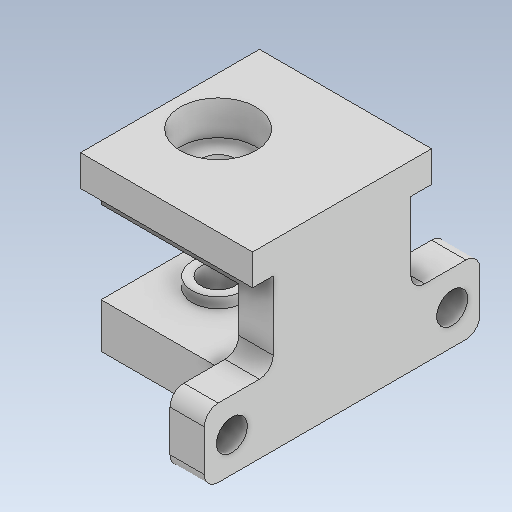
# Autodesk Inventor part: 10-03-024
Saved by Autodesk Inventor 2020 (Build 240168000, 168)
## iProperties
Created: 2019-11-02
Part Number: 10-03-024
Material: Generic
Document SubType Name: Modeling
Designer: iuliu
Density: 1 g/cm^3
Appearance: Default
Description: Intinzator X
Mass: 9.36931 g
Surface Area: 50.6885 cm^2
Volume: 9.36931 cm^3
Author: iuliu
Subject: 012
Autodesk Inventor part; units mm, degrees
ref_plane "YZ Plane" through (0, 0, 0) normal (1, 0, 0) x (0, 1, 0)
ref_plane "XZ Plane" through (0, 0, 0) normal (0, 1, 0) x (-1, 0, 0)
ref_plane "XY Plane" through (0, 0, 0) normal (0, 0, 1) x (1, 0, 0)
sketch "Sketch1" plane through (0, 0, 0) normal (0, 0, 1) x (1, 0, 0)
  line L0 (-12.5, 12.5) -> (12.5, 12.5)
  line L1 (12.5, 12.5) -> (12.5, -12.5)
  line L2 (12.5, -12.5) -> (-12.5, -12.5)
  line L3 (-12.5, -12.5) -> (-12.5, 12.5)
  point P0 (0, 0)
  point P1 (-12.5, 0)
  point P2 (0, 12.5)
  dimension "d0" = 25
  dimension "d1" = 25
  constraints: 8 end point, 2 midpoint, 2 parallel, 1 horizontal, 1 horizontal alignment, 1 perpendicular, 1 vertical alignment
  measures "d0" distance of L2.end L0.start
  measures "d1" distance between parallel lines of L1 L3
extrude "Extrusion1" add sketch "Sketch1" along normal blind 20
sketch "Sketch2" plane through (0, 0, 20) normal (0, 0, 1) x (1, 0, 0)
  line L0 (-12.5, -6) -> (7.5, -6)
  line L1 (7.5, -6) -> (7.5, 6)
  line L2 (7.5, 6) -> (-12.5, 6)
  line L3 (-12.5, 6) -> (-12.5, -6)
  line L4 (-12.5, 12.5) -> (-12.5, -12.5) projected
  line L5 (12.5, -12.5) -> (12.5, 12.5) projected
  point P0 (0, 0)
  point P1 (7.5, 0)
  point P2 (12.5, 0)
  dimension "d4" = 12
  dimension "d5" = 5
  constraints: 8 end point, 2 midpoint, 2 parallel, 1 collinear, 1 horizontal, 1 horizontal alignment, 1 perpendicular
  measures "d4" distance of L0.end L1.end
  measures "d5" distance between parallel lines of L5 L1
extrude "Extrusion2" cut sketch "Sketch2" against normal through all
sketch "Sketch3" plane through (-12.5, -12.5, 0) normal (0, -1, 0) x (1, 0, 0)
  line L0 (0, 0) -> (0, 20) projected
  point P0 (12.5, 0)
  point P1 (7, 10)
  point P2 (0, 10)
  dimension "d8" = 7
  constraints: 1 horizontal alignment, 1 midpoint
  measures "d8" distance from line of L0 point (7, 10)
hole "Hole1" at (-5.5, -12.5, 10) direction (0, 1, 0) diameter 5 end through all
sketch "Sketch4" plane through (-12.5, 12.5, 0) normal (0, 1, 0) x (1, 0, 0)
  line L0 (25, -23) -> (0, -23)
  line L1 (0, -23) -> (0, -20)
  line L2 (0, -20) -> (25, -20)
  line L3 (25, -20) -> (25, -23)
  line L4 (25, -20) -> (0, -20) projected
  line L5 (0, 0) -> (0, -20) projected
  line L6 (25, 0) -> (25, -20) projected
  line L7 (25, 0) -> (0, 0)
  line L8 (0, 0) -> (0, 3)
  line L9 (0, 3) -> (25, 3)
  line L10 (25, 3) -> (25, 0)
  line L11 (25, 0) -> (0, 0) projected
  point P0 (12.5, 0)
  dimension "d16" = 3
  constraints: 16 end point, 7 collinear, 4 parallel, 2 horizontal, 2 perpendicular
  measures "d16" distance of L2.end L0.start
extrude "Extrusion3" add sketch "Sketch4" against normal blind 3 contours L0 L1 L2 L3 | L7 L8 L9 L10
sketch "Sketch7" plane through (12.5, -12.5, 20) normal (1, 0, 0) x (0, 0, -1)
  line L0 (-10, 0) -> (-10, 10)
  line L1 (-10, 10) -> (30, 10)
  line L2 (30, 10) -> (30, 0)
  line L3 (20, 0) -> (0, 0) projected
  line L4 (20, 0) -> (20, 22) projected
  line L5 (0, 0) -> (0, 22) projected
  circle A0 centre (26, 5) radius 2.25
  circle A1 centre (-6, 5) radius 2.25
  line L6 (20, 0) -> (0, 0) projected
  line L7 (-10, 0) -> (32.446, 0)
  point P0 (20, 12.5)
  point P1 (30, 5)
  point P2 (20, 10)
  point P3 (0, 10)
  point P4 (20, 0)
  point P5 (0, 0)
  dimension "d30" = 10
  dimension "d31" = 10
  dimension "d32" = 4.5
  dimension "d33" = 4
  dimension "d34" = 4
  dimension "d50" = 10
  dimension "d51" = 0
  constraints: 8 end point, 2 centre point, 2 horizontal alignment, 1 equal radius, 1 horizontal, 1 midpoint, 1 parallel, 1 point on line
  measures "d30" distance between parallel lines of L4 L2
  measures "d31" distance between parallel lines of L5 L0
  measures "d32" diameter of A0
  measures "d33" distance from line of L2 A0.centre
  measures "d34" distance from line of L0 A1.centre
  measures "d50" distance between parallel lines of L6 L1
  measures "d51" distance between parallel lines of L3 L7
extrude "Extrusion5" add sketch "Sketch7" against normal up to surface (5 mm away) contours L0 L1 L5 L7 | L4 L1 L2 L7
sketch "Sketch6" plane through (-12.5, 12.5, 23) normal (0, 1, 0) x (1, 0, 0)
  circle A0 centre (7, 13) radius 2.5 projected
  circle A1 centre (7, 13) radius 1.5
  point P0 (12.5, 23)
  dimension "d26" = 3
  constraints: 1 centre point, 1 coincident
  measures "d26" diameter of A1
extrude "Extrusion4" add sketch "Sketch6" against normal blind 2
sketch "Sketch8" plane through (-12.5, 12.5, 23) normal (0, 1, 0) x (1, 0, 0)
  circle A0 centre (7, 13) radius 1.5 projected
  circle A1 centre (7, 13) radius 3.75
  point P0 (12.5, 23)
  dimension "d37" = 7.5
  constraints: 1 centre point, 1 coincident
  measures "d37" diameter of A1
extrude "Extrusion6" add sketch "Sketch8" against normal up to surface (25 mm away)
sketch "Sketch9" plane through (-12.5, 12.5, 23) normal (0, 0, 1) x (1, 0, 0)
  line L0 (0, -8) -> (20, -8)
  line L1 (20, -8) -> (20, -17)
  line L2 (20, -17) -> (0, -17)
  line L3 (0, -17) -> (0, -8)
  line L4 (0, -18.5) -> (0, -25) projected
  line L5 (20, -6.5) -> (20, -18.5) projected
  line L6 (0, -6.5) -> (20, -6.5) projected
  line L7 (20, -18.5) -> (0, -18.5) projected
  point P0 (12.5, -12.5)
  point P1 (20, -15)
  dimension "d40" = 1.5
  dimension "d41" = 1.5
  constraints: 8 end point, 2 collinear, 2 parallel, 1 horizontal, 1 perpendicular
  measures "d40" distance between parallel lines of L0 L6
  measures "d41" distance between parallel lines of L7 L2
extrude "Extrusion7" cut sketch "Sketch9" against normal through all
move faces "Move2" translate (0, 1.5, 0) faces at (7, 12.5, 10)
fillet "Fillet2" radius 2 6 edges at (10, -2.5, 20) (10, -2.5, 30) (10, -12.5, 30) (10, -12.5, -10) (10, -2.5, -10) (10, -2.5, 0)
sketch "Sketch11" plane through (-12.5, 14, 23) normal (0, 1, 0) x (1, 0, 0)
  circle A0 centre (7, 13) radius 1.5 projected
  point P0 (12.5, 23)
hole "Hole3" at (-5.5, 14, 10) direction (0, -1, 0) diameter 5 end through all counterbore diameter 11 counterbore depth 5
equation "\"d30\" = d31"
body "Solid1"
